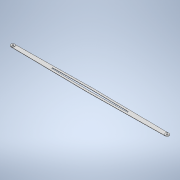
# Autodesk Inventor part: kozepso szalag 8mm
Saved by Autodesk Inventor 2020 (Build 240168000, 168)
## iProperties
Created: 2021-11-24
Part Number: kozepso szalag 8mm
Material: Generic
Document SubType Name: Modeling
Designer: Gábor
Density: 1 g/cm^3
Appearance: Default
Author: Gábor
Autodesk Inventor part; units mm, degrees
ref_plane "YZ Plane" through (0, 0, 0) normal (1, 0, 0) x (0, 1, 0)
ref_plane "XZ Plane" through (0, 0, 0) normal (0, 1, 0) x (-1, 0, 0)
ref_plane "XY Plane" through (0, 0, 0) normal (0, 0, 1) x (1, 0, 0)
sketch "Sketch1" plane through (0, 0, 0) normal (0, 1, 0) x (-1, 0, 0)
  circle A0 centre (0, 0) radius 7.5
  circle A1 centre (0, 0) radius 2.75
  line L0 (0, 0) -> (-294.76, 0)
  circle A2 centre (-294.76, 0) radius 4
  circle A3 centre (-294.76, 0) radius 11.5
  line L1 (0, 7.5) -> (-294.603914, 11.498941)
  line L2 (0, -7.5) -> (-294.603914, -11.498941)
  line L3 (-294.76, 0) -> (-296.697507, 0)
  line L4 (-296.697507, 0) -> (-296.697507, -11.527359)
  line L5 (-296.697507, -11.527359) -> (-294.76, -11.527359)
  line L6 (-294.76, -11.527359) -> (-294.76, 0)
  line L7 (0, 0) -> (-2.749747, 0.037318)
  line L8 (0, 0) -> (-2.749747, -0.037318)
  line L9 (0, 0) -> (-2.749747, -0.037318)
  line L10 (-7.5, 0) -> (-294.704301, 3.999612)
  line L11 (-7.5, 0) -> (-294.704301, -3.999612)
  circle A4 centre (-589.52, 0) radius 7.5
  circle A5 centre (-589.52, 0) radius 2.75
  line L12 (-589.52, 7.5) -> (-294.916086, 11.498941)
  line L13 (-589.52, -7.5) -> (-294.916086, -11.498941)
  line L14 (-582.02, 0) -> (-294.815699, 3.999612)
  line L15 (-582.02, 0) -> (-294.815699, -3.999612)
  dimension "d4" = 23
  dimension "d0" = 15
  dimension "d1" = 5.5
  dimension "d2" = 294.76
  dimension "d3" = 8
  constraints: 32 end point, 11 symmetric about line, 8 point on circle, 5 centre point, 5 coincident, 4 tangent, 2 horizontal, 2 parallel, 1 perpendicular, 1 point on line, 6 other
  measures "d0" diameter of A0
  measures "d1" diameter of A1
  measures "d2" distance of L0.start L0.end
  measures "d3" diameter of A2
extrude "Extrusion1" add sketch "Sketch1" along normal blind 1 contours A0 L10 A3 L1 | L2 A3 L11 A0 | A3 L10 A2 L14 | A3 L6 A2 L11 | A3 L14 A4 L12 | A3 L4 L15 A2 L6 | L13 L4 A3 | L15 L4 A3 | A3 L4 L13 A4 L15
extrude "Extrusion2" add sketch "Sketch1" along normal blind 2 contours A0 | A4
fillet "Fillet1" radius 2 2 edges at (7.5, 0.5, 0) (582.02, 0.5, 0)
body "Solid1"
